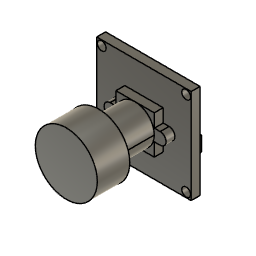
SuporteCamara (Autodesk Fusion 360 archive; units mm, degrees)
design "camera"
Autodesk Fusion 360 part; units mm, degrees
sketch "Sketch1" plane through (0, 0, 0) normal (0, 1, 0) x (1, 0, 0)
  line L0 (0, 0) -> (32, 0)
  line L1 (32, 0) -> (32, -32)
  line L2 (32, -32) -> (0, -32)
  line L3 (0, -32) -> (0, 0)
  circle A0 centre (1.6953, -30.2758) radius 1.5
  circle A1 centre (1.6953, -1.6758) radius 1.5
  circle A2 centre (30.3047, -30.2758) radius 1.5
  circle A3 centre (30.3047, -1.6758) radius 1.5
  line L4 (-1, -16) -> (38, -16)
  line L5 (0, -13) -> (9.5, -13)
  line L6 (32, -13) -> (22.5, -13)
  line L7 (9.5, 0.8661) -> (9.5, -33)
  line L8 (22.5, 0.9345) -> (22.5, -33)
  line L9 (16, 2.2342) -> (16, -35)
  line L10 (22.5, -9.5) -> (9.5, -9.5)
  line L11 (9.5, -9.5) -> (9.5, -22.5)
  line L12 (9.5, -22.5) -> (22.5, -22.5)
  line L13 (22.5, -22.5) -> (22.5, -9.5)
  line L14 (22.5, -9.5) -> (9.5, -22.5) construction
  line L15 (9.5, -9.5) -> (22.5, -22.5) construction
  circle A4 centre (16, -16) radius 6.5
  line L16 (0, 1) -> (10, 1)
  line L17 (32, 1) -> (20, 1)
  line L18 (10, 1) -> (10, -6)
  line L19 (20, 1) -> (20, -6)
  line L20 (10, -5.4961) -> (20, -5.4961)
  line L21 (20, -5.4961) -> (20, -0.4961)
  line L22 (20, -0.4961) -> (10, -0.4961)
  line L23 (10, -0.4961) -> (10, -5.4961)
  line L24 (24.5, -14) -> (22.5, -14)
  line L25 (22.5, -14) -> (22.5, -18)
  line L26 (22.5, -18) -> (24.5, -18)
  line L27 (24.5, -18) -> (24.5, -14)
  arc A5 (24.5, -18) -> (24.5, -14) centre (24.5, -16) ccw
  arc A6 (22.5, -15.9983) -> (22.5, -16.0017) centre (24.5, -16) ccw
  arc A7 (7.5, -14) -> (7.5, -18) centre (7.5, -16) ccw
  line L28 (7.5, -14) -> (9.5, -14)
  line L29 (9.5, -18) -> (7.5, -18)
  point P0 (16, -16)
  constraint horizontal L0
  constraint vertical L1
  constraint horizontal L2
  constraint vertical L3
  constraint coincident L0.start L3.end
  constraint coincident L3 L5.start
  constraint perpendicular L3 L5
  constraint coincident L1 L6.start
  constraint perpendicular L1 L6
  constraint perpendicular L2 L7
  constraint perpendicular L2 L8
  constraint perpendicular L2 L9
  constraint horizontal L10
  constraint perpendicular L10 L11
  constraint parallel L10 L12
  constraint parallel L11 L13
  constraint coincident L14 P0
  constraint coincident L15 P0
  constraint coincident L4 P0
  constraint coincident L9 P0
  constraint coincident P0 A4.centre
  constraint tangent L13 A4
  constraint perpendicular L3 L16
  constraint perpendicular L8 L17
  constraint perpendicular L0 L18
  constraint perpendicular L0 L19
  constraint horizontal L20
  constraint vertical L21
  constraint horizontal L22
  constraint vertical L23
  constraint coincident L18 L20.start
  constraint horizontal L24
  constraint vertical L25
  constraint horizontal L26
  constraint vertical L27
  constraint midpoint L27 A5.centre
  constraint coincident L8 A6.end
  constraint coincident L8 A6.start
  constraint concentric A5 A6
  constraint symmetric L9 L24.start A7.start
  constraint symmetric L9 L24.end L28.end
  constraint symmetric L9 L25.end L29.start
  constraint symmetric L9 L26.end A7.end
  constraint symmetric L9 A5 A7
extrude "Extrude1" add sketch "Sketch1" against normal blind 3
extrude "Extrude2" add sketch "Sketch1" along normal blind 12.5 contours L9 L18 L20 L22 L23 | L9 L19 L20 L21 L22
extrude "Extrude3" add sketch "Sketch1" against normal blind 6 contours L7 L10 L11 A4 | L4 L9 A4 | L8 L10 L13 A4 L25 | L4 L9 A4 | L4 L7 L11 A7 L28 | L4 L7 L11 A7 L29 | L4 L9 A4 | L4 L9 A4 | L4 L8 L13 L24 L25 L27 | L4 L8 L13 L25 L26 L27 | L8 L12 L13 A4 L25 | L7 L11 L12 A4 | L4 L27 A5 | L4 L27 A5
extrude "Extrude4" add sketch "Sketch1" against normal blind 18.4 contours L4 L9 A4 | L4 L9 A4 | L4 L9 A4 | L4 L9 A4
sketch "Sketch2" plane through (0, 0, 0) normal (0, 1, 0) x (1, 0, 0)
  circle A0 through (26.5, -16, -18.3) (10.75, -6.9067, -18.3) (10.75, -25.0933, -18.3)
extrude "Extrude5" add sketch "Sketch2" against normal blind 11 contours A0 in plane through (0, -18.3, 0) normal (0, 1, 0)
